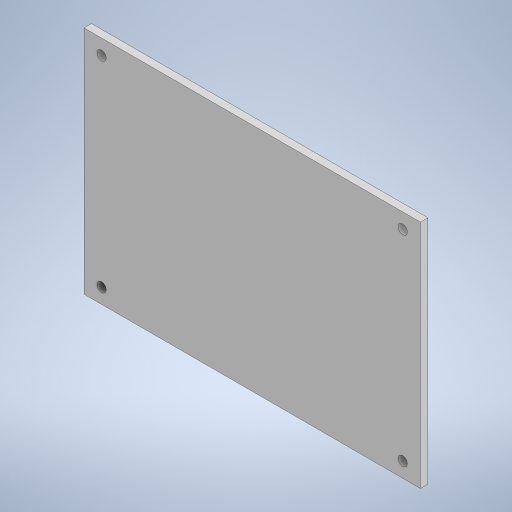
# Autodesk Inventor part: 만능기판 소형
Saved by Autodesk Inventor 2023.1 (Build 271208000, 208)
## iProperties
Created: 2022-08-14
Part Number: 만능기판 소형
Material: 일반
Document SubType Name: Modeling
Designer: fly01
Density: 1 g/cm^3
Appearance: 기본값
Author: fly01
Autodesk Inventor part; units mm, degrees
ref_plane "YZ Plane" through (0, 0, 0) normal (1, 0, 0) x (0, 1, 0)
ref_plane "XZ Plane" through (0, 0, 0) normal (0, 1, 0) x (-1, 0, 0)
ref_plane "XY Plane" through (0, 0, 0) normal (0, 0, 1) x (1, 0, 0)
sketch "스케치1" plane through (0, 0, 0) normal (0, 0, 1) x (1, 0, 0)
  line L0 (-35.8, -24.55) -> (35.8, -24.55)
  line L1 (35.8, -24.55) -> (35.8, 24.55)
  line L2 (35.8, 24.55) -> (-35.8, 24.55)
  line L3 (-35.8, 24.55) -> (-35.8, -24.55)
  line L4 (-35.8, -24.55) -> (35.8, 24.55) construction
  line L5 (35.8, -24.55) -> (-35.8, 24.55) construction
  line L6 (0, 0) -> (6.2436, 0)
  line L7 (0, 0) -> (0, 9.2645)
  circle A0 centre (-32.05, 21.35) radius 1
  circle A1 centre (32.05, 21.35) radius 1
  circle A2 centre (-32.05, -21.35) radius 1
  circle A3 centre (32.05, -21.35) radius 1
  dimension "d0" = 71.6
  dimension "d1" = 49.1
  dimension "d2" = 2
  dimension "d3" = 42.7
  dimension "d4" = 64.1
  constraints: 16 end point, 4 centre point, 3 symmetric about line, 2 horizontal, 2 midpoint, 2 parallel, 1 perpendicular, 1 vertical, 3 other
  measures "d0" distance of L2.end L1.end
  measures "d1" distance of L0.end L1.end
  measures "d2" diameter of A0
  measures "d3" distance of A2.centre A0.centre
  measures "d4" distance of A1.centre A0.centre
extrude "돌출1" add sketch "스케치1" along normal blind 1.6
